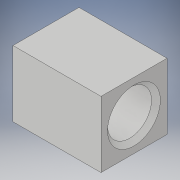
# Autodesk Inventor part: heavy lithium cell receptical
Saved by Autodesk Inventor 2019 (Build 230136000, 136)
## iProperties
Created: 2020-03-28
Part Number: heavy lithium cell receptical
Material: Generic
Document SubType Name: Modeling
Designer: q
Density: 1 g/cm^3
Appearance: Default
Author: q
Autodesk Inventor part; units mm, degrees
ref_plane "YZ Plane" through (0, 0, 0) normal (1, 0, 0) x (0, 1, 0)
ref_plane "XZ Plane" through (0, 0, 0) normal (0, 1, 0) x (-1, 0, 0)
ref_plane "XY Plane" through (0, 0, 0) normal (0, 0, 1) x (1, 0, 0)
sketch "Sketch1" plane through (0, 0, 0) normal (1, 0, 0) x (0, 1, 0)
  line L0 (0, 0) -> (750, 0)
  line L1 (750, 0) -> (750, -750)
  line L2 (750, -750) -> (0, -750)
  line L3 (0, -750) -> (0, 0)
  dimension "d0" = 750
  dimension "d1" = 750
  constraints: 8 end point, 2 parallel, 1 horizontal, 1 perpendicular
  measures "d0" distance of L1.end L2.end
  measures "d1" distance of L0.end L1.end
extrude "Extrusion1" add sketch "Sketch1" along normal blind 1000
sketch "Sketch2" plane through (1000, 0, 0) normal (1, 0, 0) x (0, 0, -1)
  line L0 (750, 0) -> (750, 750) projected
  line L1 (0, 0) -> (750, 0) projected
  circle A0 centre (374.0764, 375) radius 250
  dimension "d4" = 500
  constraints: 1 centre point
  measures "d4" diameter of A0
extrude "Extrusion2" cut sketch "Sketch2" against normal blind 750
sketch "Sketch3" plane through (250, 375, -374.0764) normal (1, 0, 0) x (0, 0, -1)
  line L0 (0, 0) -> (-100, 0)
  line L1 (0, 0) -> (100, 0)
  circle A0 centre (100, 0) radius 50
  circle A1 centre (-100, 0) radius 50
  point P0 (-374.0764, -375)
  dimension "d7" = 100
  dimension "d8" = 100
  dimension "d9" = 100
  dimension "d10" = 100
  constraints: 4 end point, 2 centre point, 2 coincident, 2 horizontal
  measures "d7" distance of L0.start L0.end
  measures "d8" distance of L0.start L1.end
  measures "d9" diameter of A0
  measures "d10" diameter of A1
extrude "Extrusion3" add sketch "Sketch3" along normal blind 50
chamfer "Chamfer1" distance 50 angle 45 1 edges at (250, 375, -124.0764)
chamfer "Chamfer2" distance 50 angle 45 1 edges at (1000, 375, -124.0764)
body "Solid1"
